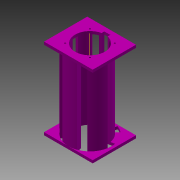
# Autodesk Inventor part: 知能ロボコン外筒
Saved by Autodesk Inventor 2013 (Build 170138000, 138)
## iProperties
Created: 2014-05-15
Part Number: 知能ロボコン外筒
Material: ABS プラスチック
Document SubType Name: Modeling
Designer: horumo136
Density: 1.06 g/cm^3
Mass: 221.773 g
Surface Area: 739.47 cm^2
Volume: 209.219 cm^3
Author: horumo136
Autodesk Inventor part; units mm, degrees
ref_plane "YZ Plane" through (0, 0, 0) normal (1, 0, 0) x (0, 1, 0)
ref_plane "XZ Plane" through (0, 0, 0) normal (0, 1, 0) x (-1, 0, 0)
ref_plane "XY Plane" through (0, 0, 0) normal (0, 0, 1) x (1, 0, 0)
sketch "スケッチ1" plane through (0, 0, 0) normal (0, 0, 1) x (1, 0, 0)
  line L0 (-45, -40) -> (45, -40)
  line L1 (45, -40) -> (45, 40)
  line L2 (45, 40) -> (-45, 40)
  line L3 (-45, 40) -> (-45, -40)
  line L4 (-45, -40) -> (45, 40) construction
  line L5 (45, -40) -> (-45, 40) construction
  point P0 (0, 0)
  dimension "d0" = 90
  dimension "d1" = 80
  constraints: 12 end point, 2 midpoint, 2 parallel, 1 horizontal, 1 perpendicular
  measures "d0" distance of L2.end L1.end
  measures "d1" distance of L1.end L0.end
extrude "押し出し1" add sketch "スケッチ1" along normal blind 5
sketch "スケッチ2" plane through (0, 0, 5) normal (0, 0, 1) x (1, 0, 0)
  circle A0 centre (0, 0) radius 40
  dimension "d4" = 80
  constraints: 1 centre point, 1 coincident
  measures "d4" diameter of A0
extrude "押し出し2" add sketch "スケッチ2" along normal blind 140
sketch "スケッチ3" plane through (0, 0, 0) normal (0, 0, -1) x (-1, 0, 0)
  circle A0 centre (0, 0) radius 27.5
  dimension "d8" = 55
  constraints: 1 centre point, 1 coincident
  measures "d8" diameter of A0
extrude "押し出し3" cut sketch "スケッチ3" against normal blind 145
sketch "スケッチ4" plane through (0, 0, 145) normal (0, 0, 1) x (1, 0, 0)
  circle A0 centre (0, 0) radius 40 projected
  line L0 (-45, 40) -> (45, 40)
  line L1 (45, 40) -> (45, -40)
  line L2 (45, -40) -> (-45, -40)
  line L3 (-45, -40) -> (-45, 40)
  line L4 (-45, 40) -> (45, -40) construction
  line L5 (45, 40) -> (-45, -40) construction
  circle A1 centre (0, 0) radius 20
  dimension "d11" = 90
  dimension "d12" = 80
  dimension "d26" = 40
  constraints: 12 end point, 2 midpoint, 2 parallel, 1 centre point, 1 coincident, 1 horizontal, 1 perpendicular
  measures "d11" distance of L1.end L2.end
  measures "d12" distance of L0.end L1.end
  measures "d26" diameter of A1
extrude "押し出し4" add sketch "スケッチ4" along normal blind 5
sketch "スケッチ5" plane through (-45, 40, 145) normal (0, 1, 0) x (1, 0, 0)
  line L0 (0, 0) -> (45, 0) projected
  line L1 (90, -5) -> (0, -5) projected
  line L2 (45, 145) -> (45, -5)
  line L3 (39.5, 0) -> (50.5, 0)
  line L4 (50.5, 0) -> (50.5, 120)
  line L5 (50.5, 120) -> (39.5, 120)
  line L6 (39.5, 120) -> (39.5, 0)
  dimension "d15" = 11
  dimension "d16" = 120
  dimension "d17" = 5.5
  constraints: 10 end point, 2 parallel, 1 horizontal, 1 midpoint, 1 perpendicular, 1 point on line
  measures "d15" distance of L5.end L4.end
  measures "d16" distance of L4.end L3.end
  measures "d17" distance between parallel lines of L6 L2
extrude "押し出し5" cut sketch "スケッチ5" against normal blind 15
sketch "スケッチ7" plane through (0, 0, 150) normal (0, 0, 1) x (1, 0, 0)
  circle A0 centre (0, 0) radius 20 projected
  line L0 (45, 40) -> (-45, 40) projected
  line L1 (-5.5, 22) -> (5.5, 22)
  line L2 (5.5, 22) -> (5.5, 32)
  line L3 (5.5, 32) -> (-5.5, 32)
  line L4 (-5.5, 32) -> (-5.5, 22)
  line L5 (0, 40) -> (0, 0)
  circle A1 centre (0, 0) radius 27.5
  dimension "d29" = 11
  dimension "d30" = 10
  dimension "d31" = 5.5
  dimension "d32" = 8
  dimension "d57" = 55
  constraints: 10 end point, 3 parallel, 1 centre point, 1 coincident, 1 horizontal, 1 midpoint, 1 perpendicular
  measures "d29" distance of L3.end L2.end
  measures "d30" distance of L2.end L1.end
  measures "d31" distance between parallel lines of L4 L5
  measures "d32" distance between parallel lines of L3 L0
  measures "d57" diameter of A1
extrude "押し出し8" cut sketch "スケッチ7" against normal blind 5 contours L1 L4 A1 L5 | L5 A1 L2 L1 | A1 L4 L3 L5 | L5 L3 L2 A1
sketch "スケッチ10" plane through (0, 0, 150) normal (0, 0, 1) x (1, 0, 0)
  circle A0 centre (0, 0) radius 20 projected
  circle A1 centre (0, 0) radius 27.5
  point P0 (-5.5, 19.2289)
  point P1 (5.5, 19.2289)
  dimension "d58" = 55
  constraints: 1 centre point, 1 coincident
  measures "d58" diameter of A1
extrude "押し出し9" cut sketch "スケッチ10" against normal blind 5 contours A0 | A1
sketch "スケッチ11" plane through (0, 0, 150) normal (0, 0, 1) x (1, 0, 0)
  arc A0 (-5.5, 26.9444) -> (5.5, 26.9444) centre (0, 0) ccw projected
  circle A1 centre (0, 0) radius 32.5
  line L0 (0, 0) -> (22.981, 22.981)
  line L1 (0, 0) -> (32.5, 0) construction
  circle A2 centre (22.981, 22.981) radius 1.5
  circle A3 centre (-22.981, 22.981) radius 1.5
  circle A4 centre (-22.981, -22.981) radius 1.5
  circle A5 centre (22.981, -22.981) radius 1.5
  dimension "d61" = 65
  dimension "d62" = 45
  dimension "d63" = 3
  dimension "d66" = 360
  constraints: 4 centre point, 4 end point, 3 coincident, 1 equal length, 1 horizontal, 12 other
  measures "d62" angle of L1 L0
  measures "d63" diameter of A2
hole "穴2" at (22.981, 22.981, 150) at (-22.981, 22.981, 150) at (-22.981, -22.981, 150) at (22.981, -22.981, 150) direction (0, 0, -1) diameter 3 depth 4.5 tip angle 118
sketch "スケッチ16" plane through (0, 0, 0) normal (0, 0, -1) x (-1, 0, 0)
  circle A0 centre (0, 0) radius 27.5 projected
  line L0 (-45, -40) -> (-45, 40) projected
  line L1 (0, 0) -> (40, 0)
  line L2 (0, 0) -> (39.3923, -6.9459)
  line L3 (0, 0) -> (40, 0) construction
  line L4 (0, 0) -> (39.3923, 6.9459)
  line L5 (0, 0) -> (25.7115, 30.6418)
  line L6 (0, 0) -> (13.6808, 37.5877)
  line L7 (0, 0) -> (-13.6808, 37.5877)
  line L8 (0, 0) -> (-25.7115, 30.6418)
  line L9 (0, 0) -> (-39.3923, 6.9459)
  line L10 (0, 0) -> (-39.3923, -6.9459)
  line L11 (0, 0) -> (-25.7115, -30.6418)
  line L12 (0, 0) -> (-13.6808, -37.5877)
  line L13 (0, 0) -> (13.6808, -37.5877)
  line L14 (0, 0) -> (25.7115, -30.6418)
  arc A1 (-39.3923, 6.9459) -> (-39.3923, -6.9459) centre (-0.5848, 0) ccw
  arc A2 (-25.7115, -30.6418) -> (-13.6808, -37.5877) centre (-0.2924, -0.5065) ccw
  arc A3 (13.6808, -37.5877) -> (25.7115, -30.6418) centre (0.2924, -0.5065) ccw
  arc A4 (39.3923, -6.9459) -> (39.3923, 6.9459) centre (0.5848, 0) ccw
  arc A5 (25.7115, 30.6418) -> (13.6808, 37.5877) centre (0.2924, 0.5065) ccw
  arc A6 (-13.6808, 37.5877) -> (-25.7115, 30.6418) centre (-0.2924, 0.5065) ccw
  dimension "d80" = 40
  dimension "d81" = 40
  dimension "d82" = 10
  dimension "d85" = 360
  dimension "d89" = 360
  constraints: 28 end point, 12 point on circle, 6 centre point, 1 coincident, 1 equal length, 1 horizontal, 1 perpendicular, 1 symmetric about line, 56 other
  measures "d80" distance of L1.start L1.end
  measures "d81" distance of L1.start L2.end
  measures "d82" angle of L2 L3
extrude "押し出し12" cut sketch "スケッチ16" against normal blind 145 contours L10 A0 L9 | A0 L10 A1 L9
pattern_circular "円形状パターン1" count 6 over 360 about axis through (0, 0, 0) along (0, 0, 1) of "押し出し12"
sketch "スケッチ18" plane through (0, 0, 5) normal (0, 0, 1) x (1, 0, 0)
  line L0 (45, 40) -> (0, 40) projected
  arc A0 (39.3923, -6.9459) -> (39.3923, 6.9459) centre (0.5848, 0) ccw projected
  arc A1 (40.009, 0) -> (0, 40) centre (0.163, 0.154) ccw
  line L1 (0, 40) -> (0, 32.5)
  line L2 (40.009, 0) -> (32.509, 0)
  line L3 (0.163, 0.154) -> (28.4473, 28.4383)
  line L4 (0.163, 0.154) -> (40.163, 0.154) construction
  line L5 (0.163, 0.154) -> (23.144, 23.135)
  arc A2 (32.509, 0) -> (0, 32.5) centre (0.5246, 0.5157) ccw
  arc A3 (0, 40) -> (-40.009, 0) centre (-0.163, 0.154) ccw
  line L6 (-40.009, 0) -> (-32.509, 0)
  arc A4 (0, 32.5) -> (-32.509, 0) centre (-0.5246, 0.5157) ccw
  dimension "d97" = 7.5
  dimension "d98" = 7.5
  dimension "d99" = 40
  dimension "d100" = 45
  dimension "d101" = 32.5
  constraints: 12 end point, 10 point on circle, 4 centre point, 4 symmetric about line, 2 perpendicular, 1 equal length, 1 horizontal, 1 point on line, 2 other
  measures "d97" distance of L0.end L1.end
  measures "d98" distance of L2.start L2.end
  measures "d99" distance of L3.start L3.end
  measures "d100" angle of L4 L3
  measures "d101" distance of L3.start L5.end
extrude "押し出し13" cut sketch "スケッチ18" along normal blind 140
